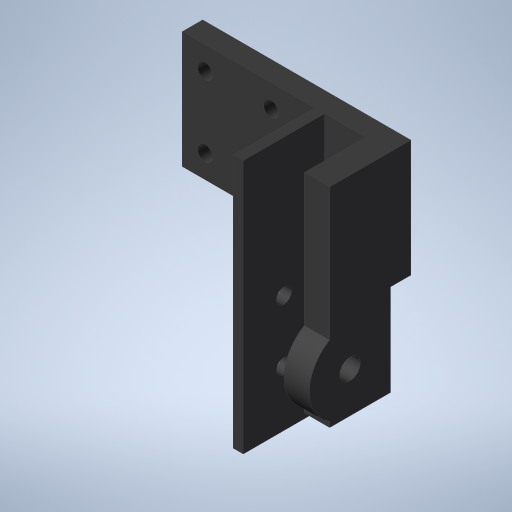
# Autodesk Inventor part: робот-энкодер
Saved by Autodesk Inventor 2024.2 (Build 282272000, 272)
## iProperties
Created: 2025-11-27
Part Number: робот-энкодер
Material: Типовые
Document SubType Name: Modeling
Designer: Zakhar
Density: 1 g/cm^3
Appearance: По умолчанию
Author: Zakhar
Autodesk Inventor part; units mm, degrees
ref_plane "YZ Plane" through (0, 0, 0) normal (1, 0, 0) x (0, 1, 0)
ref_plane "XZ Plane" through (0, 0, 0) normal (0, 1, 0) x (-1, 0, 0)
ref_plane "РабПлоскость1" through (0, 0, 0) normal (0, 0, 1) x (1, 0, 0)
sketch "Эскиз1" plane through (0, 0, 0) normal (0, 0, 1) x (1, 0, 0)
  circle A0 centre (22, -134.9569) radius 1.5
  circle A1 centre (22, -120.9569) radius 1.5
  circle A2 centre (35, -134.9569) radius 1.5
  circle A3 centre (35, -120.9569) radius 1.5
  line L0 (25.3767, -96.9033) -> (9.3929, -97.3164) projected
  line L1 (46.6684, -70.3473) -> (46.1406, -50.3565) projected
  line L2 (48, -90) -> (48, -70.3473) projected
  line L3 (17.5, -139.4569) -> (58.5, -139.4569)
  line L4 (58.5, -139.4569) -> (58.5, -116.4569)
  line L5 (58.5, -116.4569) -> (17.5, -116.4569)
  line L6 (17.5, -116.4569) -> (17.5, -139.4569)
  ellipse E0 centre (13.2497, -96.1261) end of major axis (24.2459, -95.8358) minor radius 0.1657 projected
  point P0 (0, 0)
  point P1 (12.1906, -152.9569)
  dimension "d0" = 18
  dimension "d2" = 14
  dimension "d3" = 14
  dimension "d4" = 3
  dimension "d5" = 3
  dimension "d6" = 3
  dimension "d7" = 3
  dimension "d8" = 13
  dimension "d9" = 13
  dimension "d10" = 13
  dimension "d11" = 13
  dimension "d12" = 23
  dimension "d13" = 41
  dimension "d14" = 4.5
  dimension "d15" = 4.5
  dimension "d33" = 23.5
  dimension "d34" = 23.5
  constraints: 8 end point, 4 centre point, 2 parallel, 1 horizontal, 1 perpendicular, 1 other
  measures "d0" vertical distance of point (12.191, -152.957) A0.centre
  measures "d2" distance of A0.centre A1.centre
  measures "d3" distance of A2.centre A3.centre
  measures "d4" diameter of A3
  measures "d5" diameter of A1
  measures "d6" diameter of A0
  measures "d7" diameter of A2
  measures "d8" distance from line of A2.centre L2
  measures "d9" distance of A2.centre A0.centre
  measures "d10" distance from line of L1 A3.centre
  measures "d11" distance of A3.centre A1.centre
  measures "d12" distance of L3.end L4.end
  measures "d13" distance of L4.end L5.end
  measures "d14" distance from line of L6 A0.centre
  measures "d15" distance from line of L3 A0.centre
  measures "d33" distance from line of L4 A2.centre
  measures "d34" distance from line of L4 A3.centre
extrude "Выдавливание1" add sketch "Эскиз1" along normal blind 4 contours L6 L5 L4 L3
sketch "Эскиз2" plane through (0, 0, 4) normal (0, 0, 1) x (1, 0, 0)
  line L0 (43.5, -166.4569) -> (45.5, -166.4569)
  line L1 (45.5, -166.4569) -> (45.5, -116.4569)
  line L2 (45.5, -116.4569) -> (43.5, -116.4569)
  line L3 (43.5, -116.4569) -> (43.5, -166.4569)
  line L4 (53.5, -116.4569) -> (58.5, -116.4569)
  line L5 (58.5, -116.4569) -> (58.5, -157.4569)
  line L6 (58.5, -157.4569) -> (53.5, -157.4569)
  line L7 (53.5, -157.4569) -> (53.5, -116.4569)
  line L8 (58.5, -139.4569) -> (58.5, -116.4569) projected
  line L9 (58.5, -116.4569) -> (17.5, -116.4569) projected
  line L10 (17.5, -139.4569) -> (58.5, -139.4569) projected
  point P0 (0, 0)
  point P1 (58.5, -139.4569)
  point P2 (53.5, -139.4569)
  dimension "d18" = 8
  dimension "d19" = 18
  dimension "d20" = 5
  dimension "d21" = 2
  dimension "d22" = 50
  constraints: 16 end point, 4 parallel, 3 collinear, 2 horizontal, 2 perpendicular
  measures "d18" distance between parallel lines of L1 L7
  measures "d19" distance between parallel lines of L10 L6
  measures "d20" distance between parallel lines of L5 L7
  measures "d21" distance between parallel lines of L1 L3
  measures "d22" distance of L2.end L0.start
extrude "Выдавливание2" add sketch "Эскиз2" along normal blind 12 contours L10 L5 L6 L7 | L7 L4 L5 L10
sketch "Эскиз3" plane through (53.5, -157.4569, 4) normal (-1, 0, 0) x (0, 0, 1)
  line L0 (0, 18) -> (0, 41)
  line L1 (0, 18) -> (0, -9) construction
  line L2 (0, -9) -> (6, -9) construction
  line L3 (6, 41) -> (6, -9) construction
  line L4 (0, 41) -> (6, 41)
  circle A0 centre (8, 8) radius 1.55
  line L5 (-4, 18) -> (0, 18) projected
  line L6 (12, 41) -> (12, 0) projected
  line L7 (0, 0) -> (12, 0) projected
  point P0 (-4, 157.4569)
  dimension "d26" = 3.1
  dimension "d40" = 4
  dimension "d41" = 8
  constraints: 2 end point, 1 centre point
  measures "d26" diameter of A0
  measures "d40" distance from line of L6 A0.centre
  measures "d41" distance from line of L7 A0.centre
extrude "Выдавливание3" cut sketch "Эскиз3" against normal through all
thread "Резьба1" size "M3x0.5" class "6H" standard "ANSI Metric M Profile" full length
extrude "Выдавливание4" add sketch "Эскиз2" along normal blind 16 contours L3 L10 L1 L0 | L3 L2 L1 L10
sketch "Эскиз4" plane through (58.5, -139.4569, 0) normal (1, 0, 0) x (0, 0, -1)
  circle A0 centre (-12, -10) radius 1.55 projected
  circle A1 centre (-12, -10) radius 2.05
  circle A2 centre (-12, -10) radius 8
  line L0 (-4, -18) -> (-16, -18) projected
  point P0 (0, 139.4569)
  dimension "d35" = 4.1
  constraints: 2 centre point, 2 coincident, 1 tangent
  measures "d35" diameter of A1
extrude "Выдавливание5" cut sketch "Эскиз4" against normal up to surface (5 mm away) contours A0 | A1
extrude "Выдавливание6" add sketch "Эскиз4" against normal up to surface (5 mm away) contours A2
sketch "Эскиз5" plane through (43.5, -166.4569, 4) normal (-1, 0, 0) x (0, 0, 1)
  circle A0 centre (8, 17) radius 2.05 projected
  line L0 (0, 27) -> (0, 9) projected
  line L1 (0, 9) -> (12, 9) projected
  line L2 (12, 50) -> (12, 23.9282) projected
  line L3 (0, 50) -> (12, 50) projected
  line L4 (0, 27) -> (0, 50) projected
  arc A1 (12, 10.0718) -> (12, 23.9282) centre (8, 17) ccw projected
  line L5 (12, 10.0718) -> (12, 9) projected
  line L6 (16, 17) -> (0, 17) construction
  line L7 (16, 50) -> (16, 0) projected
  circle A2 centre (8, 11) radius 1.5
  circle A3 centre (8, 23) radius 1.5
  line L8 (8, 11) -> (8, 23) construction
  line L9 (0, 9) -> (3, 9)
  line L10 (3, 9) -> (3, 24)
  line L11 (3, 24) -> (0, 24)
  line L12 (0, 24) -> (0, 9)
  point P0 (-4, 166.4569)
  point P1 (8, 17)
  point P2 (0, 24)
  point P3 (3, 9)
  dimension "d49" = 3
  dimension "d50" = 3
  dimension "d52" = 15
  dimension "d53" = 6
  dimension "d54" = 5
  dimension "d55" = 15
  constraints: 14 end point, 3 midpoint, 3 parallel, 2 centre point, 2 perpendicular, 1 horizontal, 1 point on circle, 1 point on line, 1 vertical
  measures "d49" diameter of A2
  measures "d50" diameter of A3
  measures "d53" distance of point (8, 17) L8.start
  measures "d54" distance between parallel lines of L10 L8
  measures "d55" distance of L9.end L10.end
extrude "Выдавливание7" cut sketch "Эскиз5" against normal blind 10 contours L11 L10 L1 L0 | A2 | A3
equation "\"d34\" = d33"
